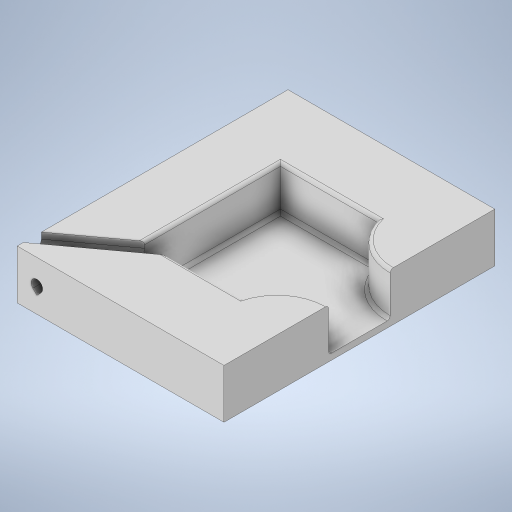
# Autodesk Inventor part: Top v2
Saved by Autodesk Inventor 2024 (Build 280153000, 153)
## iProperties
Created: 2024-02-16
Part Number: Top v2
Material: Generic
Document SubType Name: Modeling
Designer: CJ110
Density: 1 g/cm^3
Appearance: Default
Author: CJ110
Autodesk Inventor part; units mm, degrees
note: some values were not read from the file. Chosen so that the rebuilt part matches the saved one: direction of "Emboss1".
ref_plane "YZ Plane" through (0, 0, 0) normal (1, 0, 0) x (0, 1, 0)
ref_plane "XZ Plane" through (0, 0, 0) normal (0, 1, 0) x (-1, 0, 0)
sketch "Sketch1" plane through (0, 0, 0) normal (0, 1, 0) x (-1, 0, 0)
  line L0 (0, 0) -> (106.68, 0)
  line L1 (106.68, 0) -> (106.68, 139.7)
  line L2 (106.68, 139.7) -> (0, 139.7)
  line L3 (0, 139.7) -> (0, 0)
  dimension "d0" = 106.68
  dimension "d1" = 139.7
  constraints: 8 end point, 2 parallel, 1 horizontal, 1 perpendicular
  measures "d0" distance of L1.end L2.end
  measures "d1" distance of L0.end L1.end
extrude "Extrusion1" add sketch "Sketch1" along normal blind 25.4
sketch "Sketch2" plane through (0, 25.4, 0) normal (0, 1, 0) x (1, 0, 0)
  line L0 (-75.98, -100) -> (-35.78, -100)
  line L1 (-35.78, -100) -> (-35.78, -39.7)
  line L2 (-35.78, -39.7) -> (-75.98, -39.7)
  line L3 (-75.98, -39.7) -> (-75.98, -100)
  line L4 (-106.68, 0) -> (-106.68, -139.7) projected
  line L5 (-106.68, -139.7) -> (0, -139.7) projected
  line L6 (0, -139.7) -> (0, 0) projected
  line L7 (0, 0) -> (-106.68, 0) projected
  line L8 (-106.68, -69.85) -> (0, -69.85) construction
  line L9 (-53.34, -139.7) -> (-53.34, 0) construction
  line L10 (-55.88, -100) -> (-55.88, -39.7) construction
  line L11 (-30.7, -34.62) -> (-81.06, -34.62)
  line L12 (-81.06, -34.62) -> (-81.06, -105.08)
  line L13 (-81.06, -105.08) -> (-30.7, -105.08)
  line L14 (-30.7, -105.08) -> (-30.7, -34.62)
  line L15 (-30.7, -34.62) -> (-81.06, -105.08) construction
  line L16 (-81.06, -34.62) -> (-30.7, -105.08) construction
  point P0 (-75.98, -69.85)
  point P1 (-55.88, -69.85)
  dimension "d4" = 60.3
  dimension "d5" = 40.2
  dimension "d7" = 2.54
  dimension "d14" = 5.08
  dimension "d15" = 5.08
  constraints: 26 end point, 10 midpoint, 4 parallel, 2 horizontal, 2 perpendicular, 1 point on line
  measures "d4" distance of L2.end L0.start
  measures "d5" distance of L1.end L2.end
  measures "d7" distance between parallel lines of L9 L10
  measures "d14" distance between parallel lines of L12 L3
  measures "d15" distance between parallel lines of L0 L13
extrude "Extrusion2" cut sketch "Sketch2" against normal blind 22.225 contours L3 L2 L1 L0 | L14 L13 L12 L11
sketch "Sketch3" plane through (0, 25.4, 0) normal (0, 1, 0) x (1, 0, 0)
  line L0 (-106.68, 0) -> (-106.68, -139.7) projected
  line L1 (-106.68, -139.7) -> (0, -139.7) projected
  line L2 (0, -139.7) -> (0, 0) projected
  line L3 (0, 0) -> (-106.68, 0) projected
  arc A0 (-81.06, -105.08) -> (-106.68, -85.725) centre (-106.68, -112.359) ccw
  arc A1 (-106.68, -53.975) -> (-81.06, -34.62) centre (-106.68, -27.341) ccw
  line L4 (-106.68, -85.725) -> (-81.06, -85.725) construction
  line L5 (-106.68, -53.975) -> (-81.06, -53.975) construction
  line L6 (-30.7, -105.08) -> (-81.06, -105.08) projected
  line L7 (-81.06, -105.08) -> (-81.06, -34.62) projected
  line L8 (-81.06, -34.62) -> (-30.7, -34.62) projected
  line L9 (-30.7, -34.62) -> (-30.7, -105.08) projected
  line L10 (-106.68, 0) -> (-106.68, -139.7) projected
  line L11 (-106.68, -139.7) -> (0, -139.7) projected
  line L12 (0, -139.7) -> (0, 0) projected
  line L13 (0, 0) -> (-106.68, 0) projected
  dimension "d10" = 31.75
  constraints: 4 end point, 4 point on circle, 4 point on line, 2 centre point, 2 perpendicular, 2 tangent, 1 equal radius
  measures "d10" distance of L5.start L4.start
extrude "Extrusion3" cut sketch "Sketch3" against normal up to surface (22.225 mm away) contours A1 L7 A0 L0 | L8 L9 L6 L7
sketch "Sketch4" plane through (0, 0, 0) normal (0, -1, 0) x (1, 0, 0)
  circle A0 centre (-95.25, 25.4) radius 3
  circle A1 centre (-95.25, 114.3) radius 3
  line L0 (-106.68, 0) -> (-106.68, 139.7) projected
  line L1 (-106.68, 139.7) -> (0, 139.7) projected
  line L2 (0, 0) -> (-106.68, 0) projected
  dimension "d16" = 11.43
  dimension "d17" = 25.4
  dimension "d18" = 25.4
  dimension "d19" = 11.43
  dimension "d20" = 6
  constraints: 2 centre point, 1 equal radius
  measures "d16" distance from line of L0 A1.centre
  measures "d17" distance from line of L1 A1.centre
  measures "d18" distance from line of L2 A0.centre
  measures "d19" distance from line of L0 A0.centre
  measures "d20" diameter of A1
extrude "Extrusion4" cut sketch "Sketch4" against normal blind 11
ref_plane "Work Plane1" through (-106.68, 0, 69.85) normal (0, 0, 1) x (1, 0, 0)
sketch "Sketch5" plane through (-106.68, 0, 139.7) normal (0, 0, 1) x (1, 0, 0)
  line L0 (0, 0) -> (106.68, 0) projected
  line L1 (106.68, 0) -> (106.68, 25.4) projected
  line L2 (0, 25.4) -> (106.68, 25.4) projected
  line L3 (0, 0) -> (0, 25.4) projected
  line L4 (0, 12.7) -> (106.68, 12.7) construction
  circle A0 centre (96.52, 12.7) radius 3
  point P0 (106.68, 0)
  dimension "d23" = 6
  dimension "d24" = 10.16
  constraints: 2 end point, 2 midpoint, 1 centre point, 1 point on line
  measures "d23" diameter of A0
  measures "d24" distance from line of L1 A0.centre
extrude "Extrusion5" cut sketch "Sketch5" against normal blind 11 contours A0
mirror "Mirror1" about plane through (-106.68, 0, 69.85) normal (0, 0, 1) of "Extrusion5"
sketch "Sketch6" plane through (0, 0, 0) normal (0, -1, 0) x (1, 0, 0)
  circle A0 centre (-95.25, 114.3) radius 3 projected
  circle A1 centre (-95.25, 25.4) radius 3 projected
  line L0 (-106.68, 0) -> (-106.68, 139.7) projected
  line L1 (0, 0) -> (-106.68, 0) projected
  line L2 (0, 139.7) -> (0, 0) projected
  line L3 (-106.68, 139.7) -> (0, 139.7) projected
  line L4 (-53.34, 139.7) -> (-53.34, 0) construction
  line L5 (0, 69.85) -> (-106.68, 69.85) construction
  line L6 (-42.545, 109.5375) -> (-42.545, 30.1625) construction
  line L7 (-42.545, 30.1625) -> (-64.135, 30.1625) construction
  line L8 (-64.135, 30.1625) -> (-64.135, 109.5375) construction
  line L9 (-64.135, 109.5375) -> (-42.545, 109.5375) construction
  line L10 (-53.34, 109.5375) -> (-53.34, 30.1625) construction
  line L11 (-42.545, 69.85) -> (-64.135, 69.85) construction
  line L12 (-59.3702, 101.9751) -> (-47.4414, 101.9751)
  line L13 (-47.4414, 101.9751) -> (-47.3098, 100.0369)
  spline S0 degree 2 poles (-47.3098, 100.0369) (-47.3098, 98.5891) (-48.2072, 97.7396) knots 0 0 0 1 1 1
  spline S1 degree 2 poles (-48.2072, 97.7396) (-49.1165, 96.9021) (-50.5044, 96.9021) knots 0 0 0 1 1 1
  spline S2 degree 2 poles (-50.5044, 96.9021) (-52.2512, 96.9021) (-53.017, 98.4216) knots 0 0 0 1 1 1
  spline S3 degree 2 poles (-53.017, 98.4216) (-53.5673, 95.9808) (-56.1876, 95.9808) knots 0 0 0 1 1 1
  spline S4 degree 2 poles (-56.1876, 95.9808) (-57.5157, 95.9808) (-58.5087, 96.7825) knots 0 0 0 1 1 1
  spline S5 degree 2 poles (-58.5087, 96.7825) (-59.5018, 97.5961) (-59.5018, 99.4147) knots 0 0 0 1 1 1
  spline S6 degree 2 poles (-59.5018, 99.4147) (-59.5018, 100.0728) (-59.43, 100.8624) knots 0 0 0 1 1 1
  spline S7 degree 2 poles (-59.43, 100.8624) (-59.3702, 101.5564) (-59.3702, 101.9751) knots 0 0 0 1 1 1
  line L14 (-53.6152, 99.9053) -> (-53.6152, 101.0419)
  line L15 (-53.6152, 101.0419) -> (-55.6492, 101.0419)
  spline S8 degree 2 poles (-55.6492, 101.0419) (-57.7789, 101.0419) (-58.3532, 100.5753) knots 0 0 0 1 1 1
  spline S9 degree 2 poles (-58.3532, 100.5753) (-58.6523, 100.1804) (-58.6523, 99.3908) knots 0 0 0 1 1 1
  spline S10 degree 2 poles (-58.6523, 99.3908) (-58.6523, 98.0627) (-57.8866, 97.4884) knots 0 0 0 1 1 1
  spline S11 degree 2 poles (-57.8866, 97.4884) (-57.1208, 96.95) (-56.0919, 96.95) knots 0 0 0 1 1 1
  spline S12 degree 2 poles (-56.0919, 96.95) (-55.2663, 96.95) (-54.68, 97.297) knots 0 0 0 1 1 1
  spline S13 degree 2 poles (-54.68, 97.297) (-54.0818, 97.6679) (-53.8425, 98.2063) knots 0 0 0 1 1 1
  spline S14 degree 2 poles (-53.8425, 98.2063) (-53.6152, 98.7806) (-53.6152, 99.9053) knots 0 0 0 1 1 1
  line L16 (-47.4414, 102.8007) -> (-59.3702, 102.8007)
  spline S15 degree 2 poles (-59.3702, 102.8007) (-59.4061, 103.7938) (-59.5018, 105.1817) knots 0 0 0 1 1 1
  line L17 (-59.5018, 105.1817) -> (-59.2984, 105.1817)
  spline S16 degree 2 poles (-59.2984, 105.1817) (-58.9036, 103.7339) (-56.2355, 103.7339) knots 0 0 0 1 1 1
  line L18 (-56.2355, 103.7339) -> (-50.3369, 103.7339)
  spline S17 degree 2 poles (-50.3369, 103.7339) (-47.9918, 103.7339) (-47.5132, 105.1817) knots 0 0 0 1 1 1
  line L19 (-47.5132, 105.1817) -> (-47.3098, 105.1817)
  spline S18 degree 2 poles (-47.3098, 105.1817) (-47.4175, 104.0091) (-47.4414, 102.8007) knots 0 0 0 1 1 1
  line L20 (-50.5403, 101.0419) -> (-52.8136, 101.0419)
  line L21 (-52.8136, 101.0419) -> (-52.8136, 100.1685)
  spline S19 degree 2 poles (-52.8136, 100.1685) (-52.8136, 99.0797) (-52.2273, 98.4934) knots 0 0 0 1 1 1
  spline S20 degree 2 poles (-52.2273, 98.4934) (-51.641, 97.8952) (-50.5283, 97.8952) knots 0 0 0 1 1 1
  spline S21 degree 2 poles (-50.5283, 97.8952) (-49.3797, 97.8952) (-48.7815, 98.5413) knots 0 0 0 1 1 1
  spline S22 degree 2 poles (-48.7815, 98.5413) (-48.1952, 99.1754) (-48.1952, 100.0608) knots 0 0 0 1 1 1
  spline S23 degree 2 poles (-48.1952, 100.0608) (-48.1952, 100.5394) (-48.4345, 100.8385) knots 0 0 0 1 1 1
  spline S24 degree 2 poles (-48.4345, 100.8385) (-49.0447, 101.0419) (-50.5403, 101.0419) knots 0 0 0 1 1 1
  spline S25 degree 2 poles (-59.0471, 96.1842) (-57.9584, 95.1433) (-56.2474, 95.1433) knots 0 0 0 1 1 1
  spline S26 degree 2 poles (-56.2474, 95.1433) (-54.4168, 95.1433) (-53.2921, 96.2321) knots 0 0 0 1 1 1
  spline S27 degree 2 poles (-53.2921, 96.2321) (-54.0698, 94.0785) (-56.1517, 94.0785) knots 0 0 0 1 1 1
  spline S28 degree 2 poles (-56.1517, 94.0785) (-57.1807, 94.0785) (-57.9823, 94.6767) knots 0 0 0 1 1 1
  spline S29 degree 2 poles (-57.9823, 94.6767) (-58.7839, 95.2749) (-59.0471, 96.1842) knots 0 0 0 1 1 1
  spline S30 degree 2 poles (-52.658, 96.7466) (-51.7487, 96.0526) (-50.5044, 96.0526) knots 0 0 0 1 1 1
  spline S31 degree 2 poles (-50.5044, 96.0526) (-49.5233, 96.0526) (-48.7336, 96.4355) knots 0 0 0 1 1 1
  spline S32 degree 2 poles (-48.7336, 96.4355) (-47.932, 96.8423) (-47.6568, 97.3568) knots 0 0 0 1 1 1
  spline S33 degree 2 poles (-47.6568, 97.3568) (-47.8961, 96.2321) (-48.6259, 95.6339) knots 0 0 0 1 1 1
  spline S34 degree 2 poles (-48.6259, 95.6339) (-49.3558, 95.0356) (-50.2531, 95.0356) knots 0 0 0 1 1 1
  spline S35 degree 2 poles (-50.2531, 95.0356) (-51.0428, 95.0356) (-51.7487, 95.5381) knots 0 0 0 1 1 1
  spline S36 degree 2 poles (-51.7487, 95.5381) (-52.4307, 96.0287) (-52.658, 96.7466) knots 0 0 0 1 1 1
  spline S37 degree 2 poles (-53.34, 80.9412) (-55.4338, 80.9412) (-56.8696, 81.5754) knots 0 0 0 1 1 1
  spline S38 degree 2 poles (-56.8696, 81.5754) (-58.2934, 82.1975) (-58.9754, 83.3342) knots 0 0 0 1 1 1
  spline S39 degree 2 poles (-58.9754, 83.3342) (-59.6693, 84.4349) (-59.6693, 85.9186) knots 0 0 0 1 1 1
  spline S40 degree 2 poles (-59.6693, 85.9186) (-59.6693, 88.2756) (-57.9823, 89.5678) knots 0 0 0 1 1 1
  spline S41 degree 2 poles (-57.9823, 89.5678) (-56.2953, 90.86) (-53.34, 90.86) knots 0 0 0 1 1 1
  spline S42 degree 2 poles (-53.34, 90.86) (-50.2651, 90.86) (-48.6259, 89.5438) knots 0 0 0 1 1 1
  spline S43 degree 2 poles (-48.6259, 89.5438) (-47.0107, 88.2277) (-47.0107, 85.9425) knots 0 0 0 1 1 1
  spline S44 degree 2 poles (-47.0107, 85.9425) (-47.0107, 83.6333) (-48.6259, 82.2813) knots 0 0 0 1 1 1
  spline S45 degree 2 poles (-48.6259, 82.2813) (-50.2292, 80.9412) (-53.34, 80.9412) knots 0 0 0 1 1 1
  spline S46 degree 2 poles (-53.352, 82.0061) (-47.932, 82.0061) (-47.932, 85.9425) knots 0 0 0 1 1 1
  spline S47 degree 2 poles (-47.932, 85.9425) (-47.932, 89.8071) (-53.4955, 89.8071) knots 0 0 0 1 1 1
  spline S48 degree 2 poles (-53.4955, 89.8071) (-58.7241, 89.8071) (-58.7241, 85.9066) knots 0 0 0 1 1 1
  spline S49 degree 2 poles (-58.7241, 85.9066) (-58.7241, 82.0061) (-53.352, 82.0061) knots 0 0 0 1 1 1
  spline S50 degree 2 poles (-48.4943, 90.4771) (-50.4206, 91.7214) (-53.4238, 91.7214) knots 0 0 0 1 1 1
  spline S51 degree 2 poles (-53.4238, 91.7214) (-56.1397, 91.7214) (-58.1378, 90.5369) knots 0 0 0 1 1 1
  spline S52 degree 2 poles (-58.1378, 90.5369) (-56.6303, 92.8222) (-53.3161, 92.8222) knots 0 0 0 1 1 1
  spline S53 degree 2 poles (-53.3161, 92.8222) (-49.9061, 92.8222) (-48.4943, 90.4771) knots 0 0 0 1 1 1
  spline S54 degree 2 poles (-58.1977, 81.348) (-56.5226, 80.1157) (-53.1486, 80.1157) knots 0 0 0 1 1 1
  spline S55 degree 2 poles (-53.1486, 80.1157) (-50.1694, 80.1157) (-48.5063, 81.3361) knots 0 0 0 1 1 1
  spline S56 degree 2 poles (-48.5063, 81.3361) (-49.9061, 79.0149) (-53.2802, 79.0149) knots 0 0 0 1 1 1
  spline S57 degree 2 poles (-53.2802, 79.0149) (-56.6064, 79.0149) (-58.1977, 81.348) knots 0 0 0 1 1 1
  line L22 (-59.3702, 70.5559) -> (-59.3702, 70.8431)
  line L23 (-59.3702, 70.8431) -> (-47.4414, 70.8431)
  line L24 (-47.4414, 70.8431) -> (-47.4414, 66.7751)
  spline S58 degree 2 poles (-47.4414, 66.7751) (-47.4414, 65.6504) (-47.3098, 64.5736) knots 0 0 0 1 1 1
  spline S59 degree 2 poles (-47.3098, 64.5736) (-47.5252, 64.5736) (-48.0875, 64.5975) knots 0 0 0 1 1 1
  spline S60 degree 2 poles (-48.0875, 64.5975) (-48.602, 64.6334) (-49.3917, 64.6334) knots 0 0 0 1 1 1
  spline S61 degree 2 poles (-49.3917, 64.6334) (-49.8822, 64.6334) (-50.3967, 64.6932) knots 0 0 0 1 1 1
  line L25 (-50.3967, 64.6932) -> (-50.3967, 64.9684)
  spline S62 degree 2 poles (-50.3967, 64.9684) (-49.4634, 64.9923) (-48.8532, 65.4231) knots 0 0 0 1 1 1
  spline S63 degree 2 poles (-48.8532, 65.4231) (-48.2311, 65.8777) (-48.2311, 67.3374) knots 0 0 0 1 1 1
  line L26 (-48.2311, 67.3374) -> (-48.2311, 69.9098)
  line L27 (-48.2311, 69.9098) -> (-56.3312, 69.9098)
  spline S64 degree 2 poles (-56.3312, 69.9098) (-57.731, 69.9098) (-58.425, 69.515) knots 0 0 0 1 1 1
  spline S65 degree 2 poles (-58.425, 69.515) (-59.1309, 69.1202) (-59.2984, 68.2946) knots 0 0 0 1 1 1
  line L28 (-59.2984, 68.2946) -> (-59.5018, 68.2946)
  spline S66 degree 2 poles (-59.5018, 68.2946) (-59.3702, 70.2927) (-59.3702, 70.5559) knots 0 0 0 1 1 1
  line L29 (-47.4414, 75.4136) -> (-47.4414, 71.6806)
  line L30 (-47.4414, 71.6806) -> (-59.3702, 71.6806)
  line L31 (-59.3702, 71.6806) -> (-59.3702, 72.0276)
  spline S67 degree 2 poles (-59.3702, 72.0276) (-59.3702, 72.7574) (-59.5018, 74.2171) knots 0 0 0 1 1 1
  line L32 (-59.5018, 74.2171) -> (-59.2984, 74.2171)
  spline S68 degree 2 poles (-59.2984, 74.2171) (-59.0591, 73.2839) (-58.3412, 72.9249) knots 0 0 0 1 1 1
  spline S69 degree 2 poles (-58.3412, 72.9249) (-57.6234, 72.5899) (-55.9603, 72.5899) knots 0 0 0 1 1 1
  line L33 (-55.9603, 72.5899) -> (-48.2311, 72.5899)
  line L34 (-48.2311, 72.5899) -> (-48.2311, 75.4734)
  spline S70 degree 2 poles (-48.2311, 75.4734) (-48.2311, 76.5741) (-48.6857, 77.0288) knots 0 0 0 1 1 1
  spline S71 degree 2 poles (-48.6857, 77.0288) (-49.1404, 77.4835) (-50.3967, 77.7826) knots 0 0 0 1 1 1
  line L35 (-50.3967, 77.7826) -> (-50.3967, 78.0458)
  spline S72 degree 2 poles (-50.3967, 78.0458) (-50.2411, 78.0578) (-50.0736, 78.0578) knots 0 0 0 1 1 1
  spline S73 degree 2 poles (-50.0736, 78.0578) (-49.8463, 78.0578) (-49.4993, 78.0099) knots 0 0 0 1 1 1
  spline S74 degree 2 poles (-49.4993, 78.0099) (-48.2909, 77.8783) (-47.3098, 77.8783) knots 0 0 0 1 1 1
  spline S75 degree 2 poles (-47.3098, 77.8783) (-47.3816, 77.2801) (-47.4055, 76.3827) knots 0 0 0 1 1 1
  line L36 (-47.4055, 76.3827) -> (-47.4414, 75.4136)
  line L37 (-59.3702, 56.306) -> (-59.3702, 56.5931)
  line L38 (-59.3702, 56.5931) -> (-47.4414, 56.5931)
  line L39 (-47.4414, 56.5931) -> (-47.4414, 52.5252)
  spline S76 degree 2 poles (-47.4414, 52.5252) (-47.4414, 51.4005) (-47.3098, 50.3237) knots 0 0 0 1 1 1
  spline S77 degree 2 poles (-47.3098, 50.3237) (-47.5252, 50.3237) (-48.0875, 50.3476) knots 0 0 0 1 1 1
  spline S78 degree 2 poles (-48.0875, 50.3476) (-48.602, 50.3835) (-49.3917, 50.3835) knots 0 0 0 1 1 1
  spline S79 degree 2 poles (-49.3917, 50.3835) (-49.8822, 50.3835) (-50.3967, 50.4433) knots 0 0 0 1 1 1
  line L40 (-50.3967, 50.4433) -> (-50.3967, 50.7185)
  spline S80 degree 2 poles (-50.3967, 50.7185) (-49.4634, 50.7424) (-48.8532, 51.1731) knots 0 0 0 1 1 1
  spline S81 degree 2 poles (-48.8532, 51.1731) (-48.2311, 51.6278) (-48.2311, 53.0875) knots 0 0 0 1 1 1
  line L41 (-48.2311, 53.0875) -> (-48.2311, 55.6599)
  line L42 (-48.2311, 55.6599) -> (-56.3312, 55.6599)
  spline S82 degree 2 poles (-56.3312, 55.6599) (-57.731, 55.6599) (-58.425, 55.2651) knots 0 0 0 1 1 1
  spline S83 degree 2 poles (-58.425, 55.2651) (-59.1309, 54.8702) (-59.2984, 54.0447) knots 0 0 0 1 1 1
  line L43 (-59.2984, 54.0447) -> (-59.5018, 54.0447)
  spline S84 degree 2 poles (-59.5018, 54.0447) (-59.3702, 56.0428) (-59.3702, 56.306) knots 0 0 0 1 1 1
  line L44 (-47.4414, 61.1636) -> (-47.4414, 57.4307)
  line L45 (-47.4414, 57.4307) -> (-59.3702, 57.4307)
  line L46 (-59.3702, 57.4307) -> (-59.3702, 57.7776)
  spline S85 degree 2 poles (-59.3702, 57.7776) (-59.3702, 58.5075) (-59.5018, 59.9672) knots 0 0 0 1 1 1
  line L47 (-59.5018, 59.9672) -> (-59.2984, 59.9672)
  spline S86 degree 2 poles (-59.2984, 59.9672) (-59.0591, 59.0339) (-58.3412, 58.675) knots 0 0 0 1 1 1
  spline S87 degree 2 poles (-58.3412, 58.675) (-57.6234, 58.34) (-55.9603, 58.34) knots 0 0 0 1 1 1
  line L48 (-55.9603, 58.34) -> (-48.2311, 58.34)
  line L49 (-48.2311, 58.34) -> (-48.2311, 61.2235)
  spline S88 degree 2 poles (-48.2311, 61.2235) (-48.2311, 62.3242) (-48.6857, 62.7789) knots 0 0 0 1 1 1
  spline S89 degree 2 poles (-48.6857, 62.7789) (-49.1404, 63.2335) (-50.3967, 63.5327) knots 0 0 0 1 1 1
  line L50 (-50.3967, 63.5327) -> (-50.3967, 63.7959)
  spline S90 degree 2 poles (-50.3967, 63.7959) (-50.2411, 63.8078) (-50.0736, 63.8078) knots 0 0 0 1 1 1
  spline S91 degree 2 poles (-50.0736, 63.8078) (-49.8463, 63.8078) (-49.4993, 63.76) knots 0 0 0 1 1 1
  spline S92 degree 2 poles (-49.4993, 63.76) (-48.2909, 63.6284) (-47.3098, 63.6284) knots 0 0 0 1 1 1
  spline S93 degree 2 poles (-47.3098, 63.6284) (-47.3816, 63.0301) (-47.4055, 62.1328) knots 0 0 0 1 1 1
  line L51 (-47.4055, 62.1328) -> (-47.4414, 61.1636)
  line L52 (-59.3702, 40.728) -> (-53.34, 40.728)
  line L53 (-53.34, 40.728) -> (-47.4414, 46.3873)
  line L54 (-47.4414, 46.3873) -> (-47.4414, 46.0642)
  spline S94 degree 2 poles (-47.4414, 46.0642) (-47.4414, 44.7242) (-47.3098, 43.2765) knots 0 0 0 1 1 1
  line L55 (-47.3098, 43.2765) -> (-47.5132, 43.2765)
  spline S95 degree 2 poles (-47.5132, 43.2765) (-47.7046, 43.9465) (-48.1473, 43.9465) knots 0 0 0 1 1 1
  spline S96 degree 2 poles (-48.1473, 43.9465) (-48.7336, 43.9465) (-50.1454, 42.5945) knots 0 0 0 1 1 1
  line L56 (-50.1454, 42.5945) -> (-52.646, 40.2015)
  line L57 (-52.646, 40.2015) -> (-50.0378, 37.9641)
  spline S97 degree 2 poles (-50.0378, 37.9641) (-49.1643, 37.2223) (-48.4704, 37.2223) knots 0 0 0 1 1 1
  spline S98 degree 2 poles (-48.4704, 37.2223) (-47.6927, 37.2223) (-47.5132, 38) knots 0 0 0 1 1 1
  line L58 (-47.5132, 38) -> (-47.3098, 38)
  spline S99 degree 2 poles (-47.3098, 38) (-47.3098, 37.7249) (-47.3936, 36.6241) knots 0 0 0 1 1 1
  spline S100 degree 2 poles (-47.3936, 36.6241) (-47.4414, 36.1575) (-47.4414, 35.7985) knots 0 0 0 1 1 1
  spline S101 degree 2 poles (-47.4414, 35.7985) (-47.4414, 35.6071) (-47.3098, 33.8124) knots 0 0 0 1 1 1
  line L59 (-47.3098, 33.8124) -> (-47.5132, 33.8124)
  spline S102 degree 2 poles (-47.5132, 33.8124) (-47.7645, 34.6619) (-48.2072, 35.1883) knots 0 0 0 1 1 1
  spline S103 degree 2 poles (-48.2072, 35.1883) (-48.6498, 35.7028) (-49.4395, 36.3609) knots 0 0 0 1 1 1
  spline S104 degree 2 poles (-49.4395, 36.3609) (-49.4993, 36.3968) (-49.6429, 36.5164) knots 0 0 0 1 1 1
  line L60 (-49.6429, 36.5164) -> (-53.4836, 39.8067)
  line L61 (-53.4836, 39.8067) -> (-56.3551, 39.8067)
  spline S105 degree 2 poles (-56.3551, 39.8067) (-58.9754, 39.8067) (-59.2984, 38.1795) knots 0 0 0 1 1 1
  line L62 (-59.2984, 38.1795) -> (-59.5018, 38.1795)
  spline S106 degree 2 poles (-59.5018, 38.1795) (-59.3702, 40.2494) (-59.3702, 40.3212) knots 0 0 0 1 1 1
  line L63 (-59.3702, 40.3212) -> (-59.3702, 40.728)
  line L64 (-47.4414, 47.4641) -> (-53.663, 41.6014)
  line L65 (-53.663, 41.6014) -> (-59.3702, 41.6014)
  line L66 (-59.3702, 41.6014) -> (-59.3702, 41.8646)
  spline S107 degree 2 poles (-59.3702, 41.8646) (-59.3702, 42.8577) (-59.5018, 44.1379) knots 0 0 0 1 1 1
  line L67 (-59.5018, 44.1379) -> (-59.2984, 44.1379)
  spline S108 degree 2 poles (-59.2984, 44.1379) (-59.1309, 43.3961) (-58.5566, 42.9654) knots 0 0 0 1 1 1
  spline S109 degree 2 poles (-58.5566, 42.9654) (-57.9943, 42.5466) (-56.403, 42.5466) knots 0 0 0 1 1 1
  line L68 (-56.403, 42.5466) -> (-53.9263, 42.5466)
  line L69 (-53.9263, 42.5466) -> (-50.1215, 46.148)
  spline S110 degree 2 poles (-50.1215, 46.148) (-47.9679, 48.2059) (-47.5132, 49.869) knots 0 0 0 1 1 1
  line L70 (-47.5132, 49.869) -> (-47.3098, 49.869)
  spline S111 degree 2 poles (-47.3098, 49.869) (-47.4414, 48.9238) (-47.4414, 47.835) knots 0 0 0 1 1 1
  line L71 (-47.4414, 47.835) -> (-47.4414, 47.4641)
  dimension "d27" = 21.59
  dimension "d28" = 79.375
  constraints: 8 end point, 8 midpoint, 2 collinear, 1 horizontal, 2 other
  measures "d27" distance of L8.end L6.start
  measures "d28" distance of L6.start L6.end
emboss "Emboss1" sketch "Sketch6" operation cut depth 0.4 direction (0, 1, 0) contours L12 L13 S0 S1 S2 S3 S4 S5 S6 S7 | L16 S15 L17 S16 L18 S17 L19 S18 | S25 S26 S27 S28 S29 | S30 S31 S32 S33 S34 S35 S36 | S37 S38 S39 S40 S41 S42 S43 S44 S45 | S50 S51 S52 S53 | S54 S55 S56 S57 | L22 L23 L24 S58 S59 S60 S61 L25 S62 S63 L26 L27 S64 S65 L28 S66 | L29 L30 L31 S67 L32 S68 S69 L33 L34 S70 S71 L35 S72 S73 S74 S75 L36 | L37 L38 L39 S76 S77 S78 S79 L40 S80 S81 L41 L42 S82 S83 L43 S84 | L44 L45 L46 S85 L47 S86 S87 L48 L49 S88 S89 L50 S90 S91 S92 S93 L51 | L52 L53 L54 S94 L55 S95 S96 L56 L57 S97 S98 L58 S99 S100 S101 L59 S102 S103 S104 L60 L61 S105 L62 S106 L63 | L64 L65 L66 S107 L67 S108 S109 L68 L69 S110 L70 S111 L71
fillet "Fillet1" radius 1.5875 10 edges at (-30.7, 25.4, 69.85) (-55.88, 25.4, 105.08) (-90.6254, 25.4, 91.1077) (-90.6254, 25.4, 48.5923) (-55.88, 25.4, 34.62) (-55.88, 3.175, 105.08) (-30.7, 3.175, 69.85) (-55.88, 3.175, 34.62) (-90.6254, 3.175, 91.1077) (-90.6254, 3.175, 48.5923)
sketch "Sketch8" plane through (0, 25.4, 0) normal (0, 1, 0) x (1, 0, 0)
  arc A0 (-106.68, -52.3875) -> (-82.2888, -33.0325) centre (-106.68, -27.341) ccw projected
  line L0 (-29.1125, -33.0325) -> (-82.2888, -33.0325) projected
  line L1 (-29.1125, -106.6675) -> (-29.1125, -33.0325) projected
  line L2 (-82.2888, -106.6675) -> (-29.1125, -106.6675) projected
  arc A1 (-82.2888, -106.6675) -> (-106.68, -87.3125) centre (-106.68, -112.359) ccw projected
  line L3 (-106.68, -87.3125) -> (-106.68, -139.7) projected
  line L4 (-106.68, -139.7) -> (0, -139.7) projected
  line L5 (0, -139.7) -> (0, 0) projected
  line L6 (0, 0) -> (-106.68, 0) projected
  line L7 (-106.68, 0) -> (-106.68, -52.3875) projected
  arc A2 (-106.68, -55.5625) -> (-79.8875, -36.2075) centre (-106.68, -27.341) ccw projected
  line L8 (-106.68, -84.1375) -> (-106.68, -55.5625) projected
  arc A3 (-79.8875, -103.4925) -> (-106.68, -84.1375) centre (-106.68, -112.359) ccw projected
  line L9 (-32.2875, -103.4925) -> (-79.8875, -103.4925) projected
  line L10 (-32.2875, -36.2075) -> (-32.2875, -103.4925) projected
  line L11 (-79.8875, -36.2075) -> (-32.2875, -36.2075) projected
  line L12 (-32.2875, -36.2075) -> (0, -12.5001)
  line L13 (0, -3.175) -> (-44.9875, -36.2075)
  dimension "d32" = 12.7
  dimension "d33" = 3.175
  constraints: 4 end point, 3 point on line, 1 parallel
  measures "d32" distance of L13.end L10.start
  measures "d33" distance of point (0, 0) L13.start
extrude "Extrusion6" cut sketch "Sketch8" against normal blind 6.35 contours L13 L5 L12 L1 L0 | L0 L1 L12 L11 L13
fillet "Fillet2" radius 3.175 2 edges at (-21.4127, 19.05, 18.8975) (-15.35, 19.05, 23.771)
sketch "Sketch9" plane through (0, 0, 0) normal (0, 0, -1) x (-1, 0, 0)
  circle A0 centre (10.16, 12.7) radius 3 projected
  line L0 (0, 0) -> (106.68, 0) projected
  line L1 (106.68, 0) -> (106.68, 25.4) projected
  line L2 (0, 25.4) -> (106.68, 25.4) projected
  line L3 (0, 0) -> (0, 25.4) projected
  line L4 (10.16, 12.7) -> (10.16, 8.4574) construction
  line L5 (10.16, 8.4574) -> (8.0387, 10.5787)
  line L6 (10.16, 8.4574) -> (12.2813, 10.5787)
  circle A1 centre (10.16, 12.7) radius 3 projected
  constraints: 6 end point, 2 point on circle, 2 tangent, 1 perpendicular, 1 vertical
extrude "Extrusion7" cut sketch "Sketch9" against normal up to surface (11 mm away) contours A0 L6 L5
mirror "Mirror2" about plane through (-106.68, 0, 69.85) normal (0, 0, 1) of "Extrusion7"
sketch "Sketch10" plane through (0, 0, 139.7) normal (1, 0, 0) x (0, 0, -1)
  line L0 (0, 25.4) -> (127.1999, 25.4) projected
  line L1 (0, 0) -> (0, 25.4) projected
  line L2 (0, 0) -> (139.7, 0) projected
  line L3 (139.7, 0) -> (139.7, 25.4) projected
  arc A0 (127, 0) -> (107.95, 19.05) centre (107.95, 0) ccw
  arc A1 (31.75, 19.05) -> (12.7, 0) centre (31.75, 0) ccw
  line L4 (107.95, 19.05) -> (31.75, 19.05)
  line L5 (0, 0) -> (139.7, 0) projected
  line L6 (69.85, 0) -> (69.85, 25.4) construction
  line L7 (127.1999, 22.225) -> (127.1999, 25.4) projected
  line L8 (136.525, 25.4) -> (139.7, 25.4) projected
  line L9 (136.525, 25.4) -> (136.525, 22.225) projected
  ellipse E0 centre (132.586, 22.225) end of major axis (136.525, 22.225) minor radius 3.175 (132.586, 19.05) -> (136.525, 22.225) ccw projected
  line L10 (132.586, 19.05) -> (131.1389, 19.05) projected
  ellipse E1 centre (131.1389, 22.225) end of major axis (127.1999, 22.225) minor radius 3.175 (127.1999, 22.225) -> (131.1389, 19.05) ccw projected
  point P0 (69.85, 19.05)
  dimension "d40" = 114.3
  dimension "d41" = 6.35
  constraints: 6 point on line, 4 end point, 4 point on circle, 2 centre point, 2 midpoint, 1 equal radius, 1 horizontal, 1 perpendicular, 1 tangent, 2 other
  measures "d40" distance of A1.end A0.start
  measures "d41" distance between parallel lines of L0 L4
extrude "Extrusion8" cut sketch "Sketch10" against normal blind 25.4 contours A1 L4 A0 L2
fillet "Fillet4" radius 6.35 3 edges at (-25.4, 13.4704, 18.2796) (-25.4, 13.4704, 121.4204) (-25.4, 19.05, 69.85)
fillet "Fillet5" radius 3.175 5 edges at (-23.5401, 0, 125.1401) (-9.525, 0, 127) (-23.5401, 0, 14.5599) (-9.525, 0, 12.7) (-25.4, 0, 69.85)
equation "\"d18\" = d17"
equation "\"d19\" = d16"
body "Solid1"
